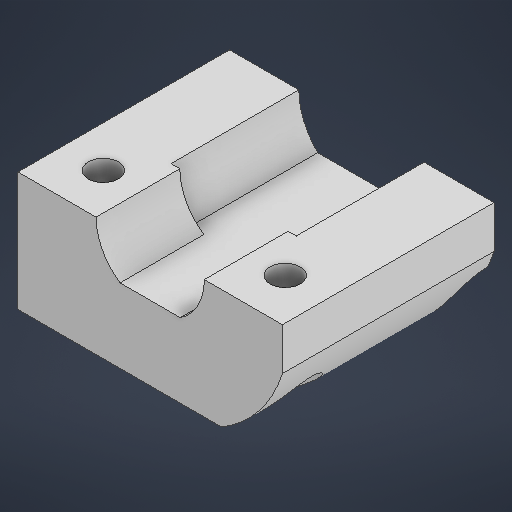
# Autodesk Inventor part: body-motor_comparment
Saved by Autodesk Inventor 2025 (Build 290162000, 162)
## iProperties
Created: 2024-10-24
Part Number: body-motor_comparment
Material: Všeobecné
Document SubType Name: Modeling
Designer: Simak
Density: 1 g/cm^3
Appearance: Výchozí
Author: Simak
Autodesk Inventor part; units mm, degrees
ref_plane "YZ Plane" through (0, 0, 0) normal (1, 0, 0) x (0, 1, 0)
ref_plane "XZ Plane" through (0, 0, 0) normal (0, 1, 0) x (-1, 0, 0)
ref_plane "XY Plane" through (0, 0, 0) normal (0, 0, 1) x (1, 0, 0)
sketch "Náčrt1" plane through (0, 0, 0) normal (0, 0, 1) x (1, 0, 0)
  line L0 (-15, 13.5) -> (-15, 0)
  line L1 (-15, 0) -> (15, 0)
  line L2 (15, 0) -> (15, 13.5)
  line L3 (15, 13.5) -> (6.1386, 13.5)
  line L4 (-6.1386, 13.5) -> (-15, 13.5)
  line L5 (-3.4165, 8.4) -> (3.4165, 8.4)
  arc A0 (3.4165, 8.4) -> (6.1386, 13.5) centre (0, 13.5) ccw
  arc A1 (-6.1386, 13.5) -> (-3.4165, 8.4) centre (0, 13.5) ccw
  arc A2 (8.1125, 0) -> (15, 8.6977) centre (0, 13.5) ccw
  point P0 (0, 0)
  point P1 (0, 0)
  dimension "d2" = 13.5
  dimension "d4" = 6.833
  dimension "d5" = 5.1
  dimension "d6" = 30
  dimension "d7" = 31.5
  constraints: 12 end point, 6 point on circle, 4 point on line, 3 centre point, 3 coincident, 3 perpendicular, 2 horizontal, 1 collinear, 1 concentric, 1 horizontal alignment, 1 midpoint, 1 vertical, 1 vertical alignment
  measures "d2" distance of L0.start L0.end
  measures "d4" distance of L5.start L5.end
  measures "d5" distance between parallel lines of L3 L5
  measures "d6" distance of L0.end L1.end
  measures "d7" diameter of A2
extrude "Vysunutí1" add sketch "Náčrt1" along normal blind 24 contours L4 A1 L5 A0 L3 L2 A2 L1 L0
sketch "Náčrt2" plane through (0, 0, 0) normal (0, 0, -1) x (-1, 0, 0)
  line L0 (15, 0) -> (-8.1125, 0) projected
  line L1 (15, 13.5) -> (15, 0) projected
  line L2 (6.1386, 13.5) -> (15, 13.5) projected
  arc A0 (3.4165, 8.4) -> (6.1386, 13.5) centre (0, 13.5) ccw projected
  line L3 (-3.4165, 8.4) -> (3.4165, 8.4) projected
  arc A1 (-6.1386, 13.5) -> (-3.4165, 8.4) centre (0, 13.5) ccw projected
  line L4 (-15, 13.5) -> (-6.1386, 13.5) projected
  line L5 (-15, 8.6977) -> (-15, 13.5) projected
  arc A2 (-15, 8.6977) -> (-8.1125, 0) centre (0, 13.5) ccw projected
  arc A3 (-7.0682, 13.5) -> (-4.8938, 8.4) centre (0, 13.5) ccw
  arc A4 (4.995, 8.4) -> (7.1386, 13.5) centre (0, 13.5) ccw
  line L6 (-15, 13.5) -> (-6.1386, 13.5) projected
  line L7 (-3.4165, 8.4) -> (-4.8938, 8.4)
  line L8 (-3.4165, 8.4) -> (3.4165, 8.4) projected
  line L9 (3.4165, 8.4) -> (4.995, 8.4)
  point P0 (0, 0)
  dimension "d11" = 1
  dimension "d12" = 0.9296
  constraints: 4 end point, 4 point on circle, 3 point on line, 2 centre point, 1 horizontal
  measures "d11" distance of L2.start A4.end
  measures "d12" distance of A3.start L4.end
extrude "Vysunutí2" cut sketch "Náčrt2" against normal blind 14.5 contours A4 L9 A0 L2 | L4 A1 L7 A3
sketch "Náčrt3" plane through (-15, 13.5, 24) normal (0, 1, 0) x (1, 0, 0)
  circle A0 centre (25.3125, 5) radius 1.7
  circle A1 centre (4.6875, 5) radius 1.7
  line L0 (8.8614, 0) -> (0, 0) projected
  line L1 (21.1386, 9.5) -> (21.1386, 0) projected
  line L2 (25.3125, 5) -> (21.1386, 0) construction
  line L3 (8.8614, 0) -> (4.6875, 5) construction
  point P0 (15, 24)
  dimension "d15" = 5
  dimension "d16" = 20.625
  dimension "d17" = 3.4
  constraints: 4 end point, 2 centre point, 1 equal length, 1 equal radius, 1 horizontal alignment
  measures "d15" distance from line of L0 L3.end
  measures "d16" distance of L3.end L2.start
  measures "d17" diameter of A1
extrude "Vysunutí3" cut sketch "Náčrt3" against normal through all
sketch "Náčrt4" plane through (-15, 0, 0) normal (0, -1, 0) x (1, 0, 0)
  circle A0 centre (25.3125, 19) radius 3
  circle A1 centre (25.3125, 19) radius 1.7 projected
  circle A2 centre (4.6875, 19) radius 1.7 projected
  circle A3 centre (4.6875, 19) radius 3
  point P0 (15, 0)
  dimension "d20" = 6
  constraints: 2 centre point, 1 coincident, 1 equal radius, 1 horizontal alignment, 2 other
  measures "d20" diameter of A0
extrude "Vysunutí4" cut sketch "Náčrt4" against normal blind 8.5 contours A0 | A1
extrude "Vysunutí5" cut sketch "Náčrt4" against normal blind 2 contours A2 | A3
sketch "Náčrt5" plane through (10.3125, 8.5, 19) normal (0, -1, 0) x (1, 0, 0)
  circle A0 centre (0, 0) radius 3 projected
  point P0 (-10.3125, -19)
  point P1 (1.4743, -2.6128)
  point P2 (-1.4743, -2.6128)
  constraints: 1 coincident
hole "Díra1" at (10.3125, 8.5, 19) direction (0, 1, 0) diameter 3.4 end through all countersink diameter 6 countersink angle 90
sketch "Náčrt7" plane through (-10.3125, 2, 19) normal (0, -1, 0) x (1, 0, 0)
  circle A0 centre (0, 0) radius 3 projected
  point P0 (10.3125, -19)
  constraints: 1 coincident
hole "Díra3" at (-10.3125, 2, 19) direction (0, 1, 0) diameter 3.4 end through all countersink diameter 6 countersink angle 90
sketch "Náčrt9" plane through (15, 8.6977, 0) normal (1, 0, 0) x (0, 0, -1)
  circle A0 centre (0, -4.8977) radius 3
  line L0 (0, -8.6977) -> (-16.9604, -8.6977) projected
  dimension "d46" = 6
  dimension "d47" = 0.8
  constraints: 1 centre point, 1 vertical alignment
  measures "d46" diameter of A0
  measures "d47" distance edge to line of A0 L0
extrude "Vysunutí6" cut sketch "Náčrt9" against normal blind 15
sketch "Náčrt10" plane through (15, 8.6977, 0) normal (1, 0, 0) x (0, 0, -1)
  line L0 (0, -1.8977) -> (0, -7.8977) projected
  arc A0 (0, -1.8977) -> (0, -7.8977) centre (0, -4.8977) ccw projected
  circle A1 centre (0, -4.8977) radius 1.95
  circle A2 centre (0, -4.8977) radius 1.75
  point P0 (0, -8.6977)
  point P1 (0, -6.6477)
  point P2 (0, -3.1477)
  point P3 (0, -2.9477)
  point P4 (0, -6.8477)
  dimension "d50" = 3.9
  dimension "d51" = 3.5
  constraints: 2 centre point, 2 coincident
  measures "d50" diameter of A1
  measures "d51" diameter of A2
extrude "Vysunutí7" cut sketch "Náčrt10" against normal through all contours L0 A2 picked at (-0.8669, -4.2091)
extrude "Vysunutí8" cut sketch "Náčrt10" against normal blind 28.5 contours L0 A2 A1 | L0 A2 picked at (-1.8696, -4.968) picked at (-0.8669, -4.2091)
